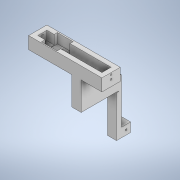
# Autodesk Inventor part: ArmAcrossPrint
Saved by Autodesk Inventor 2020 (Build 240168000, 168)
## iProperties
Created: 2020-01-21
Part Number: ArmAcrossPrint
Material: Generic
Document SubType Name: Modeling
Designer: tdmp4
Density: 1 g/cm^3
Appearance: Default
Author: tdmp4
Autodesk Inventor part; units mm, degrees
ref_plane "YZ Plane" through (0, 0, 0) normal (1, 0, 0) x (0, 1, 0)
ref_plane "XZ Plane" through (0, 0, 0) normal (0, 1, 0) x (-1, 0, 0)
ref_plane "XY Plane" through (0, 0, 0) normal (0, 0, 1) x (1, 0, 0)
sketch "Sketch1" plane through (0, 0, 0) normal (0, 1, 0) x (-1, 0, 0)
  line L0 (0, 0) -> (152.4, 0)
  line L1 (152.4, 0) -> (152.4, -38.1)
  line L2 (152.4, -38.1) -> (0, -38.1)
  line L3 (0, -38.1) -> (0, 0)
  dimension "d0" = 152.4
  dimension "d1" = 38.1
  constraints: 8 end point, 2 parallel, 1 horizontal, 1 perpendicular
  measures "d0" distance of L1.end L2.end
  measures "d1" distance of L2.end L0.start
extrude "Extrusion1" add sketch "Sketch1" along normal blind 25.4
sketch "Sketch3" plane through (0, 25.4, 0) normal (0, 1, 0) x (1, 0, 0)
  line L0 (-152.4, 0) -> (0, 0) projected
  line L1 (0, 0) -> (-9.525, 0)
  line L2 (-9.525, 0) -> (-9.525, 9.525)
  line L3 (-9.525, 9.525) -> (0, 9.525)
  line L4 (0, 9.525) -> (0, 0)
  line L5 (0, 38.1) -> (-152.4, 38.1) projected
  line L6 (-152.4, 38.1) -> (-142.875, 38.1)
  line L7 (-142.875, 38.1) -> (-142.875, 28.575)
  line L8 (-142.875, 28.575) -> (-152.4, 28.575)
  line L9 (-152.4, 28.575) -> (-152.4, 38.1)
  line L10 (-9.525, 9.525) -> (-142.875, 9.525)
  line L11 (-142.875, 9.525) -> (-142.875, 28.575)
  line L12 (-142.875, 28.575) -> (-9.525, 28.575)
  line L13 (-9.525, 28.575) -> (-9.525, 9.525)
  dimension "d4" = 9.525
  dimension "d5" = 9.525
  dimension "d6" = 9.525
  dimension "d7" = 9.525
  constraints: 24 end point, 6 parallel, 3 horizontal, 3 perpendicular
  measures "d4" distance of L2.end L3.end
  measures "d5" distance of L1.end L2.end
  measures "d6" distance of L7.end L8.end
  measures "d7" distance of L6.end L7.end
extrude "Extrusion2" cut sketch "Sketch3" against normal blind 19.05 contours L10 L11 L12 L13
sketch "Sketch4" plane through (0, 0, 0) normal (1, 0, 0) x (0, 0, -1)
  circle A0 centre (19.05, 21.5294) radius 1.7907
  circle A1 centre (19.05, 13.1683) radius 1.7907
  point P0 (0, 0)
  dimension "d24" = 3.5814
  dimension "d25" = 3.5814
  constraints: 2 centre point
  measures "d24" diameter of A0
  measures "d25" diameter of A1
extrude "Extrusion3" cut sketch "Sketch4" against normal blind 192.0875
sketch "Sketch5" plane through (0, 6.35, 0) normal (0, 1, 0) x (1, 0, 0)
  line L0 (0, 0) -> (0, 38.1) projected
  line L1 (0, 19.05) -> (-152.4, 19.05)
  line L2 (-152.4, 38.1) -> (-152.4, 0) projected
  circle A0 centre (-112.3138, 19.05) radius 9.779
  circle A1 centre (-122.0928, 19.05) radius 1.7907
  circle A2 centre (-102.5348, 19.05) radius 1.7907
  circle A3 centre (-112.3138, 29.2997) radius 1.7907
  circle A4 centre (-112.3138, 9.271) radius 1.7907
  dimension "d31" = 19.558
  dimension "d32" = 3.5814
  dimension "d33" = 3.5814
  dimension "d34" = 3.5814
  dimension "d35" = 3.5814
  constraints: 5 centre point, 3 point on circle, 3 point on line, 2 end point, 2 midpoint
  measures "d31" diameter of A0
  measures "d32" diameter of A1
  measures "d33" diameter of A2
  measures "d34" diameter of A3
  measures "d35" diameter of A4
extrude "Extrusion4" cut sketch "Sketch5" against normal blind 192.0875 contours A2 A0 L1 | L1 A0 A2 | A0 A2 L1 | L1 A2 A0 | A3 A0 | A0 A3 | A4 A0 | A0 A4 | A1 A0 L1 | L1 A0 A1 | A0 A1 L1 | L1 A1 A0
sketch "Sketch6" plane through (0, 25.4, 0) normal (0, 1, 0) x (1, 0, 0)
  line L0 (-95.0511, 1.8932) -> (-127.7029, 1.8932)
  line L1 (-127.7029, 1.8932) -> (-127.7029, 35.2854)
  line L2 (-127.7029, 35.2854) -> (-95.0511, 35.2854)
  line L3 (-95.0511, 35.2854) -> (-95.0511, 1.8932)
  point P0 (0, 0)
  constraints: 8 end point, 2 parallel, 1 horizontal, 1 perpendicular
extrude "Extrusion5" cut sketch "Sketch6" against normal blind 20.32
sketch "Sketch7" plane through (0, 0, 0) normal (0, -1, 0) x (1, 0, 0)
  line L0 (0, -38.1) -> (-152.4, -38.1) projected
  line L1 (-152.4, 0) -> (0, 0) projected
  line L2 (-55.8622, -38.1) -> (-62.2122, -38.1)
  line L3 (-62.2122, -38.1) -> (-62.2122, 0)
  line L4 (-62.2122, 0) -> (-55.8622, 0)
  line L5 (-55.8622, 0) -> (-55.8622, -38.1)
  dimension "d36" = 6.35
  constraints: 8 end point, 2 parallel, 2 point on line, 1 horizontal, 1 perpendicular
  measures "d36" distance of L3.end L4.end
extrude "Extrusion6" add sketch "Sketch7" along normal blind 58.42
sketch "Sketch8" plane through (0, 25.4, -38.1) normal (0, 0, -1) x (-1, 0, 0)
  line L0 (62.2122, -25.4) -> (62.2122, -83.82) projected
  line L1 (55.8622, -25.4) -> (55.8622, -83.82) projected
  line L2 (62.2122, -83.82) -> (55.8622, -83.82)
  line L3 (55.8622, -83.82) -> (55.8622, -58.1066)
  line L4 (55.8622, -58.1066) -> (62.2122, -58.1066)
  line L5 (62.2122, -58.1066) -> (62.2122, -83.82)
  point P0 (0, -25.4)
  constraints: 8 end point, 2 parallel, 1 horizontal, 1 perpendicular, 1 point on line
extrude "Extrusion7" add sketch "Sketch8" along normal blind 45.72
sketch "Sketch9" plane through (0, -58.42, 0) normal (0, -1, 0) x (1, 0, 0)
  line L0 (-62.2122, 0) -> (-62.2122, -83.82) projected
  line L1 (-55.8622, 0) -> (-55.8622, -83.82) projected
  line L2 (-62.2122, -83.82) -> (-55.8622, -83.82)
  line L3 (-55.8622, -83.82) -> (-55.8622, -77.4887)
  line L4 (-55.8622, -77.4887) -> (-62.2122, -77.4887)
  line L5 (-62.2122, -77.4887) -> (-62.2122, -83.82)
  point P0 (0, 0)
  constraints: 8 end point, 2 parallel, 1 horizontal, 1 perpendicular, 1 point on line
extrude "Extrusion8" add sketch "Sketch9" along normal blind 76.2
fillet "Fillet1" radius 1.5875 1 edges at (-59.0372, -58.42, -77.4887)
sketch "Sketch10" plane through (-55.8622, 0, 0) normal (1, 0, 0) x (0, 0, -1)
  line L0 (38.1, -32.7066) -> (83.82, -32.7066) projected
  line L1 (83.82, -32.7066) -> (38.1, 0)
  line L2 (38.1, 0) -> (38.1, -32.7066)
  line L3 (38.1, -32.7066) -> (83.82, -32.7066)
  point P0 (0, 0)
  constraints: 6 end point, 1 collinear, 1 perpendicular
extrude "Extrusion9" add sketch "Sketch10" against normal blind 6.35
sketch "Sketch11" plane through (-55.8622, -58.42, 0) normal (1, 0, 0) x (0, 0, -1)
  line L0 (83.82, 25.7134) -> (83.82, -76.2) projected
  line L1 (0, 0) -> (83.82, 0)
  line L2 (83.82, 0) -> (83.82, 25.7134)
  line L3 (83.82, 25.7134) -> (0, 25.7134)
  line L4 (0, 25.7134) -> (0, 0)
  line L5 (0, 58.42) -> (38.1, 58.42) projected
  line L6 (0, 58.42) -> (38.1, 58.42)
  line L7 (38.1, 58.42) -> (38.1, 25.7134)
  line L8 (38.1, 25.7134) -> (0, 25.7134)
  line L9 (0, 25.7134) -> (0, 58.42)
  line L10 (77.4887, -1.5875) -> (77.4887, -76.2) projected
  line L11 (83.82, 0) -> (77.4887, 0)
  line L12 (77.4887, 0) -> (77.4887, -76.2)
  line L13 (77.4887, -76.2) -> (83.82, -76.2)
  line L14 (83.82, -76.2) -> (83.82, 0)
  arc A0 (77.4887, -1.5875) -> (75.9012, 0) centre (75.9012, -1.5875) ccw projected
  arc A1 (77.4887, -1.5875) -> (75.9012, 0) centre (75.9012, -1.5875) ccw
  line L15 (38.1, 58.42) -> (83.82, 25.7134) projected
  line L16 (38.1, 58.42) -> (83.82, 25.7134)
  constraints: 26 end point, 7 equal length, 3 horizontal, 3 perpendicular, 2 point on circle, 1 centre point, 1 concentric, 1 point on line
extrude "Extrusion10" add sketch "Sketch11" along normal blind 12.7
sketch "Sketch14" plane through (0, -134.62, 0) normal (0, -1, 0) x (1, 0, 0)
  line L0 (-62.2122, -38.1) -> (-62.2122, -83.82) projected
  line L1 (-43.1622, -83.82) -> (-43.1622, -38.1) projected
  line L2 (-62.2122, -83.82) -> (-43.1622, -83.82)
  line L3 (-43.1622, -83.82) -> (-43.1622, -77.4782)
  line L4 (-43.1622, -77.4782) -> (-62.2122, -77.4782)
  line L5 (-62.2122, -77.4782) -> (-62.2122, -83.82)
  point P0 (0, 0)
  constraints: 8 end point, 2 parallel, 1 horizontal, 1 perpendicular, 1 point on line
extrude "Extrusion13" add sketch "Sketch14" along normal blind 11.3284
sketch "Sketch15" plane through (0, 25.4, -83.82) normal (0, 0, -1) x (-1, 0, 0)
  line L0 (43.1622, -171.3484) -> (62.2122, -171.3484) projected
  line L1 (62.2122, -171.3484) -> (43.1622, -171.3484)
  line L2 (43.1622, -171.3484) -> (43.1622, -152.2984)
  line L3 (43.1622, -152.2984) -> (62.2122, -152.2984)
  line L4 (62.2122, -152.2984) -> (62.2122, -171.3484)
  point P0 (0, -25.4)
  dimension "d57" = 19.05
  dimension "d58" = 19.05
  constraints: 8 end point, 2 parallel, 1 horizontal, 1 perpendicular
  measures "d57" distance of L1.end L2.end
  measures "d58" distance of L2.end L3.end
extrude "Extrusion14" add sketch "Sketch15" along normal blind 19.05
sketch "Sketch16" plane through (-43.1622, -58.42, 0) normal (1, 0, 0) x (0, 0, -1)
  line L0 (83.82, -68.4784) -> (102.87, -68.4784) projected
  line L1 (77.4782, -87.5284) -> (102.87, -87.5284) projected
  line L2 (83.82, -68.4784) -> (102.87, -87.5284)
  line L3 (102.87, -87.5284) -> (102.87, -68.4784) projected
  line L4 (102.87, -87.5284) -> (102.87, -68.4784)
  line L5 (102.87, -68.4784) -> (83.82, -87.5284)
  circle A0 centre (93.345, -78.0034) radius 1.7907
  point P0 (0, 58.42)
  dimension "d61" = 3.5814
  constraints: 6 end point, 1 centre point, 1 collinear, 1 midpoint
  measures "d61" diameter of A0
extrude "Extrusion15" cut sketch "Sketch16" against normal blind 39.6875 contours A0 L5 L2 | L2 L5 A0 | A0 L2 L5 | L2 A0 L5
sketch "Sketch17" plane through (-62.2122, -60.0075, -77.4887) normal (0, 0, 1) x (1, 0, 0)
  line L0 (0, -74.6125) -> (0, -85.9409) projected
  line L1 (19.05, 1.5875) -> (19.05, 0) projected
  line L2 (0, -85.9409) -> (19.05, -85.9409)
  line L3 (19.05, -85.9409) -> (19.05, 0)
  line L4 (19.05, 0) -> (0, 0)
  line L5 (0, 0) -> (0, -85.9409)
  point P0 (62.2122, 60.0075)
  constraints: 8 end point, 2 parallel, 1 horizontal, 1 perpendicular
extrude "Extrusion16" add sketch "Sketch17" along normal blind 3.9624
body "Solid1"
